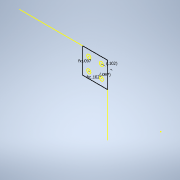
# Autodesk Inventor part: spacer1
Saved by Autodesk Inventor 2022 (Build 260153000, 153)
## iProperties
Created: 2021-06-14
Part Number: spacer1
Material: Generic
Document SubType Name: Modeling
Designer: capta
Density: 1 g/cm^3
Appearance: Default
Author: capta
Autodesk Inventor part; units mm, degrees
ref_plane "YZ Plane" through (0, 0, 0) normal (1, 0, 0) x (0, 1, 0)
ref_plane "XZ Plane" through (0, 0, 0) normal (0, 1, 0) x (-1, 0, 0)
ref_plane "XY Plane" through (0, 0, 0) normal (0, 0, 1) x (1, 0, 0)
sketch "Sketch1" plane through (0, 0, 0) normal (0, 0, 1) x (1, 0, 0)
  line L0 (-21.5598, -13.7472) -> (-21.5598, 14.1928)
  line L1 (-21.5598, 14.1928) -> (-57.1198, 14.1928)
  line L2 (-21.5598, 14.1928) -> (-31.5778, 14.1928)
  line L3 (-31.5778, 14.1928) -> (-31.5778, 3.9428)
  line L4 (-31.5778, 3.9428) -> (-21.5598, 3.9428)
  line L5 (-21.5598, 3.9428) -> (-21.5598, 14.1928)
  circle A0 centre (-24.0288, 11.6078) radius 0.85
  circle A1 centre (-29.1088, 6.5278) radius 0.85
  circle A2 centre (-24.0288, 6.5278) radius 0.85
  circle A3 centre (-29.1088, 11.6078) radius 0.85
  circle A4 centre (-26.5688, 9.0678) radius 0.6
  point P0 (0, 0)
extrude "Extrusion1" add sketch "Sketch1" along normal blind 7.1351
equation "\"d1\" = d0"
equation "\"d3\" = d2"
equation "\"d0\" = 2.585"
equation "\"d2\" = 2.469"
body "Solid1"
